Spacer (Plastic) (Autodesk Fusion 360 design; units mm, degrees)
Autodesk Fusion 360 part; units mm, degrees
sketch "sketch 165" plane through (0, 0, 0) normal (1, 0, 0) x (0, 1, 0)
  circle A0 centre (0, 0) radius 4.064
  circle A1 centre (0, 0) radius 2.1209
extrude "Extrude1" add sketch "sketch 165" along normal blind 4.8
fillet "Fillet1" radius 0.508 1 edges at (4.8, -3.789, -1.4696)
